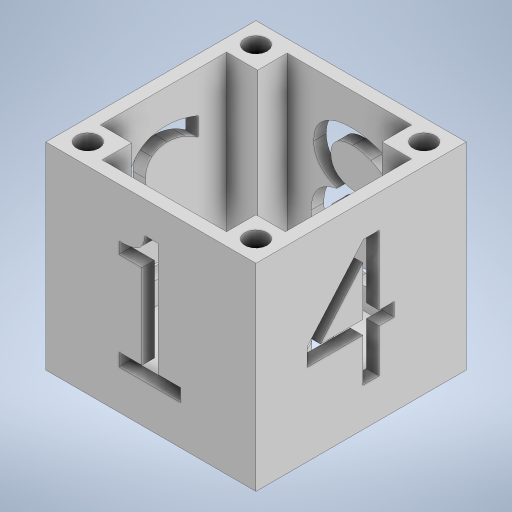
# Autodesk Inventor part: Box
Saved by Autodesk Inventor 2023 (Build 270158000, 158)
## iProperties
Created: 2023-12-17
Part Number: Box
Material: Generic
Document SubType Name: Modeling
Designer: Mustapha
Density: 1 g/cm^3
Appearance: Default
Author: Mustapha
Autodesk Inventor part; units mm, degrees
ref_plane "YZ Plane" through (0, 0, 0) normal (1, 0, 0) x (0, 1, 0)
ref_plane "XZ Plane" through (0, 0, 0) normal (0, 1, 0) x (-1, 0, 0)
ref_plane "XY Plane" through (0, 0, 0) normal (0, 0, 1) x (1, 0, 0)
sketch "Sketch1" plane through (0, 0, 0) normal (0, 1, 0) x (-1, 0, 0)
  line L0 (0, 0) -> (50, 0)
  line L1 (50, 0) -> (50, -50)
  line L2 (50, -50) -> (0, -50)
  line L3 (0, -50) -> (0, 0)
  dimension "d0" = 50
  dimension "d1" = 50
  constraints: 8 end point, 2 parallel, 1 horizontal, 1 perpendicular
  measures "d0" distance of L0.start L0.end
  measures "d1" distance of L2.end L0.start
extrude "Extrusion1" add sketch "Sketch1" along normal blind 3
sketch "Sketch2" plane through (0, 3, 0) normal (0, 1, 0) x (1, 0, 0)
  line L0 (0, 50) -> (-50, 50) projected
  line L1 (0, 50) -> (-50, 50)
  line L2 (-50, 50) -> (-50, 0)
  line L3 (-50, 0) -> (0, 0)
  line L4 (0, 0) -> (0, 50)
  line L5 (-10, 47) -> (-39.5847, 47)
  line L6 (-47, 40) -> (-47, 10)
  line L7 (-39.5847, 3) -> (-10, 3)
  line L8 (-3, 10) -> (-3, 40)
  line L9 (0, 0) -> (0, 50) projected
  line L10 (0, 50) -> (-10, 50)
  line L11 (-10, 50) -> (-10, 40)
  line L12 (-10, 40) -> (0, 40)
  line L13 (0, 40) -> (0, 50)
  line L14 (0, 25) -> (-50, 25)
  line L15 (-50, 50) -> (-50, 0) projected
  line L16 (-24.7923, 0) -> (-24.7923, 50.7224)
  line L17 (0, 0) -> (-10, 0)
  line L18 (-10, 0) -> (-10, 10)
  line L19 (-10, 10) -> (0, 10)
  line L20 (0.4153, 0) -> (-49.5847, 0)
  line L21 (-49.5847, 50) -> (-39.5847, 50)
  line L22 (-39.5847, 50) -> (-39.5847, 40)
  line L23 (-39.5847, 40) -> (-49.5847, 40)
  line L24 (-39.5847, 10) -> (-49.5847, 10)
  line L25 (-39.5847, 0) -> (-39.5847, 10)
  point P0 (-24.7923, 3)
  dimension "d10" = 3
  dimension "d11" = 3
  dimension "d12" = 3
  dimension "d13" = 3
  dimension "d14" = 10
  dimension "d15" = 10
  constraints: 46 end point, 12 symmetric about line, 8 point on line, 6 parallel, 4 perpendicular, 3 horizontal, 2 midpoint
  measures "d10" distance between parallel lines of L3 L7
  measures "d11" distance between parallel lines of L0 L5
  measures "d12" distance between parallel lines of L4 L8
  measures "d13" distance between parallel lines of L6 L2
  measures "d14" distance between parallel lines of L11 L13
  measures "d15" distance of L10.end L11.end
extrude "Extrusion2" add sketch "Sketch2" along normal blind 44 contours L4 L12 L11 L0 | L11 L5 L16 L0 | L4 L14 L8 L12 | L16 L5 L22 L0 | L4 L19 L8 L14 | L22 L23 L6 L14 L2 L0 | L4 L3 L18 L19 | L6 L24 L25 L3 L2 L14 | L16 L3 L25 L7 | L7 L18 L3 L16
sketch "Sketch3" plane through (-50, 0, 0) normal (0, 0, 1) x (1, 0, 0)
  line L0 (12.8681, 39.4555) -> (44.0571, 39.4555) construction
  line L1 (44.0571, 39.4555) -> (44.0571, 9.9644) construction
  line L2 (44.0571, 9.9644) -> (12.8681, 9.9644) construction
  line L3 (12.8681, 9.9644) -> (12.8681, 39.4555) construction
  line L4 (32.0496, 9.3582) -> (17.4143, 9.3582)
  line L5 (17.4143, 9.3582) -> (17.4143, 12.4214)
  line L6 (17.4143, 12.4214) -> (22.86, 12.4214)
  line L7 (22.86, 12.4214) -> (22.86, 32.5268)
  line L8 (22.86, 32.5268) -> (17.4143, 32.5268)
  line L9 (17.4143, 32.5268) -> (17.4143, 35.274)
  spline S0 degree 2 poles (17.4143, 35.274) (20.5018, 35.274) (23.4191, 37.0244) (23.6136, 39.4555) knots 0 0 0 1 2 2 2
  line L10 (23.6136, 39.4555) -> (26.7254, 39.4555)
  line L11 (26.7254, 39.4555) -> (26.7254, 12.4214)
  line L12 (26.7254, 12.4214) -> (32.0496, 12.4214)
  line L13 (32.0496, 12.4214) -> (32.0496, 9.3582)
  point P0 (50, 0)
  constraints: 2 other
extrude "Extrusion3" cut sketch "Sketch3" against normal blind 44
sketch "Sketch6" plane through (0, 47, 0) normal (0, 1, 0) x (1, 0, 0)
  circle A0 centre (-5, 45) radius 2.65
  line L0 (0, 0) -> (0, 50) projected
  line L1 (0, 50) -> (-50, 50) projected
  line L2 (0, 0) -> (0, 50) projected
  line L3 (0, 25) -> (-54.5112, 25)
  line L4 (0, 50) -> (-50, 50) projected
  line L5 (-25, 50) -> (-25, 0)
  circle A1 centre (-5, 5) radius 2.65
  circle A2 centre (-45, 45) radius 2.65
  circle A3 centre (-45, 5) radius 2.65
  dimension "d18" = 5
  dimension "d19" = 5
  dimension "d20" = 5.3
  dimension "d21" = 25
  constraints: 4 centre point, 4 end point, 3 symmetric about line, 2 midpoint, 1 horizontal, 1 perpendicular, 3 other
  measures "d18" distance from line of L0 A0.centre
  measures "d19" distance from line of L1 A0.centre
  measures "d20" diameter of A0
  measures "d21" distance between parallel lines of L0 L5
extrude "Extrusion4" cut sketch "Sketch6" against normal blind 5 contours A0 | A1 | A2 | A3
sketch "Sketch7" plane through (-50, 0, -50) normal (-1, 0, 0) x (0, 0, 1)
  line L0 (13.901, 39.0556) -> (42.5878, 39.0556) construction
  line L1 (42.5878, 39.0556) -> (42.5878, 7.5091) construction
  line L2 (42.5878, 7.5091) -> (13.901, 7.5091) construction
  line L3 (13.901, 7.5091) -> (13.901, 39.0556) construction
  line L4 (34.5899, 8.4235) -> (16.0891, 8.4235)
  line L5 (16.0891, 8.4235) -> (16.0891, 12.678)
  spline S0 degree 2 poles (16.0891, 12.678) (18.0826, 14.5499) (21.632, 18.0264) (23.3338, 19.8984) knots 0 0 0 1 2 2 2
  spline S1 degree 2 poles (23.3338, 19.8984) (26.7617, 23.6666) (29.2657, 28.1885) (29.2657, 30.5953) knots 0 0 0 1 2 2 2
  spline S2 degree 2 poles (29.2657, 30.5953) (29.2657, 31.8595) (28.4878, 33.7558) (27.7827, 34.3636) knots 0 0 0 1 2 2 2
  spline S3 degree 2 poles (27.7827, 34.3636) (27.0777, 34.9713) (25.2301, 35.5791) (24.1117, 35.5791) knots 0 0 0 1 2 2 2
  spline S4 degree 2 poles (24.1117, 35.5791) (23.0421, 35.5791) (20.854, 35.0443) (19.8573, 34.631) knots 0 0 0 1 2 2 2
  spline S5 degree 2 poles (19.8573, 34.631) (19.0064, 34.2906) (17.4262, 33.3182) (16.9399, 32.9778) knots 0 0 0 1 2 2 2
  line L6 (16.9399, 32.9778) -> (16.7211, 32.9778)
  line L7 (16.7211, 32.9778) -> (16.7211, 37.2566)
  spline S6 degree 2 poles (16.7211, 37.2566) (17.961, 37.8644) (22.41, 39.0556) (24.4035, 39.0556) knots 0 0 0 1 2 2 2
  spline S7 degree 2 poles (24.4035, 39.0556) (28.6093, 39.0556) (33.35, 34.6067) (33.35, 30.8141) knots 0 0 0 1 2 2 2
  spline S8 degree 2 poles (33.35, 30.8141) (33.35, 29.0394) (32.5234, 26.0734) (31.7941, 24.8093) knots 0 0 0 1 2 2 2
  spline S9 degree 2 poles (31.7941, 24.8093) (31.0647, 23.4965) (28.9497, 20.9195) (27.7827, 19.6796) knots 0 0 0 1 2 2 2
  spline S10 degree 2 poles (27.7827, 19.6796) (25.8865, 17.6132) (21.243, 13.1885) (19.8573, 11.9) knots 0 0 0 1 2 2 2
  line L8 (19.8573, 11.9) -> (34.5899, 11.9)
  line L9 (34.5899, 11.9) -> (34.5899, 8.4235)
  point P0 (50, 0)
  constraints: 2 other
extrude "Extrusion5" cut sketch "Sketch7" against normal blind 5
sketch "Sketch8" plane through (0, 0, -50) normal (0, 0, -1) x (-1, 0, 0)
  line L0 (13.682, 39.2957) -> (44.0571, 39.2957) construction
  line L1 (44.0571, 39.2957) -> (44.0571, 5.0686) construction
  line L2 (44.0571, 5.0686) -> (13.682, 5.0686) construction
  line L3 (13.682, 5.0686) -> (13.682, 39.2957) construction
  spline S0 degree 2 poles (23.9656, 35.8192) (22.8716, 35.8192) (20.7079, 35.2843) (19.6625, 34.871) knots 0 0 0 1 2 2 2
  spline S1 degree 2 poles (19.6625, 34.871) (18.6901, 34.4577) (17.2557, 33.5825) (16.6966, 33.1935) knots 0 0 0 1 2 2 2
  line L4 (16.6966, 33.1935) -> (16.4535, 33.1935)
  line L5 (16.4535, 33.1935) -> (16.4535, 37.448)
  spline S2 degree 2 poles (16.4535, 37.448) (17.7663, 38.153) (22.2638, 39.2957) (24.2817, 39.2957) knots 0 0 0 1 2 2 2
  spline S3 degree 2 poles (24.2817, 39.2957) (26.3238, 39.2957) (29.3627, 38.4691) (30.6026, 37.5939) knots 0 0 0 1 2 2 2
  spline S4 degree 2 poles (30.6026, 37.5939) (31.9154, 36.6457) (33.2768, 33.8986) (33.2768, 32.0509) knots 0 0 0 1 2 2 2
  spline S5 degree 2 poles (33.2768, 32.0509) (33.2768, 29.5712) (30.0191, 25.8273) (27.7338, 25.341) knots 0 0 0 1 2 2 2
  line L6 (27.7338, 25.341) -> (27.7338, 25.0493)
  spline S6 degree 2 poles (27.7338, 25.0493) (28.682, 24.8548) (30.8457, 23.9796) (31.7695, 23.1044) knots 0 0 0 1 2 2 2
  spline S7 degree 2 poles (31.7695, 23.1044) (32.6933, 22.2535) (33.8603, 19.5307) (33.8603, 17.5615) knots 0 0 0 1 2 2 2
  spline S8 degree 2 poles (33.8603, 17.5615) (33.8603, 15.5436) (32.4745, 12.1157) (31.2103, 10.8029) knots 0 0 0 1 2 2 2
  spline S9 degree 2 poles (31.2103, 10.8029) (29.8975, 9.4415) (26.1779, 8.0315) (23.8197, 8.0315) knots 0 0 0 1 2 2 2
  spline S10 degree 2 poles (23.8197, 8.0315) (21.5588, 8.0315) (17.1342, 9.1255) (15.6269, 9.8791) knots 0 0 0 1 2 2 2
  line L7 (15.6269, 9.8791) -> (15.6269, 14.1336)
  line L8 (15.6269, 14.1336) -> (15.9186, 14.1336)
  spline S11 degree 2 poles (15.9186, 14.1336) (17.1828, 13.2098) (21.4616, 11.508) (23.5766, 11.508) knots 0 0 0 1 2 2 2
  spline S12 degree 2 poles (23.5766, 11.508) (24.8165, 11.508) (27.2962, 12.2859) (28.1228, 13.1854) knots 0 0 0 1 2 2 2
  spline S13 degree 2 poles (28.1228, 13.1854) (28.9251, 14.085) (29.776, 16.2243) (29.776, 17.8532) knots 0 0 0 1 2 2 2
  spline S14 degree 2 poles (29.776, 17.8532) (29.776, 19.482) (28.8278, 21.5971) (27.977, 22.2049) knots 0 0 0 1 2 2 2
  spline S15 degree 2 poles (27.977, 22.2049) (27.1261, 22.8127) (24.8165, 23.2746) (23.4551, 23.2746) knots 0 0 0 1 2 2 2
  line L9 (23.4551, 23.2746) -> (21.7533, 23.2746)
  line L10 (21.7533, 23.2746) -> (21.7533, 26.6052)
  line L11 (21.7533, 26.6052) -> (23.0904, 26.6052)
  spline S16 degree 2 poles (23.0904, 26.6052) (25.7889, 26.6052) (29.1925, 29.1822) (29.1925, 31.6376) knots 0 0 0 1 2 2 2
  spline S17 degree 2 poles (29.1925, 31.6376) (29.1925, 32.7803) (28.3173, 34.4091) (27.6123, 34.8953) knots 0 0 0 1 2 2 2
  spline S18 degree 2 poles (27.6123, 34.8953) (26.8586, 35.4059) (25.011, 35.8192) (23.9656, 35.8192) knots 0 0 0 1 2 2 2
  point P0 (0, 0)
  constraints: 2 other
extrude "Extrusion6" cut sketch "Sketch8" against normal blind 5
sketch "Sketch9" plane through (0, 0, 0) normal (1, 0, 0) x (0, 0, -1)
  line L0 (11.3547, 39.1637) -> (45.4717, 39.1637) construction
  line L1 (45.4717, 39.1637) -> (45.4717, 2.8456) construction
  line L2 (45.4717, 2.8456) -> (11.3547, 2.8456) construction
  line L3 (11.3547, 2.8456) -> (11.3547, 39.1637) construction
  line L4 (32.8458, 19.4717) -> (29.272, 19.4717)
  line L5 (29.272, 19.4717) -> (29.272, 9.1637)
  line L6 (29.272, 9.1637) -> (25.4066, 9.1637)
  line L7 (25.4066, 9.1637) -> (25.4066, 19.4717)
  line L8 (25.4066, 19.4717) -> (12.157, 19.4717)
  line L9 (12.157, 19.4717) -> (12.157, 23.7018)
  line L10 (12.157, 23.7018) -> (25.5767, 39.1637)
  line L11 (25.5767, 39.1637) -> (29.272, 39.1637)
  line L12 (29.272, 39.1637) -> (29.272, 22.705)
  line L13 (29.272, 22.705) -> (32.8458, 22.705)
  line L14 (32.8458, 22.705) -> (32.8458, 19.4717)
  line L15 (25.4066, 22.705) -> (25.4066, 34.423)
  line L16 (25.4066, 34.423) -> (15.3174, 22.705)
  line L17 (15.3174, 22.705) -> (25.4066, 22.705)
  point P0 (0, 0)
  constraints: 2 other
extrude "Extrusion7" cut sketch "Sketch9" against normal blind 5
sketch "Sketch10" plane through (0, 0, 0) normal (0, -1, 0) x (1, 0, 0)
  line L0 (-36.2764, -9.4843) -> (-5.351, -9.4843) construction
  line L1 (-5.351, -9.4843) -> (-5.351, -42.6108) construction
  line L2 (-5.351, -42.6108) -> (-36.2764, -42.6108) construction
  line L3 (-36.2764, -42.6108) -> (-36.2764, -9.4843) construction
  spline S0 degree 2 poles (-15.9037, -29.9543) (-15.9037, -32.118) (-17.2894, -35.8133) (-18.5536, -37.1747) knots 0 0 0 1 2 2 2
  spline S1 degree 2 poles (-18.5536, -37.1747) (-19.8178, -38.5361) (-23.586, -40.1164) (-25.9199, -40.1164) knots 0 0 0 1 2 2 2
  spline S2 degree 2 poles (-25.9199, -40.1164) (-28.0592, -40.1164) (-32.2408, -39.1682) (-33.7724, -38.4146) knots 0 0 0 1 2 2 2
  line L4 (-33.7724, -38.4146) -> (-33.7724, -34.1601)
  line L5 (-33.7724, -34.1601) -> (-33.4806, -34.1601)
  spline S3 degree 2 poles (-33.4806, -34.1601) (-33.0187, -34.5005) (-31.2926, -35.3757) (-30.2473, -35.7647) knots 0 0 0 1 2 2 2
  spline S4 degree 2 poles (-30.2473, -35.7647) (-29.056, -36.178) (-27.0868, -36.6399) (-25.8469, -36.6399) knots 0 0 0 1 2 2 2
  spline S5 degree 2 poles (-25.8469, -36.6399) (-24.6314, -36.6399) (-22.3461, -35.7647) (-21.5195, -34.8165) knots 0 0 0 1 2 2 2
  spline S6 degree 2 poles (-21.5195, -34.8165) (-20.7659, -33.917) (-19.9879, -31.5345) (-19.9879, -29.93) knots 0 0 0 1 2 2 2
  spline S7 degree 2 poles (-19.9879, -29.93) (-19.9879, -28.3254) (-20.8631, -26.2833) (-21.6897, -25.6026) knots 0 0 0 1 2 2 2
  spline S8 degree 2 poles (-21.6897, -25.6026) (-22.5406, -24.8489) (-25.069, -24.2169) (-26.6006, -24.2169) knots 0 0 0 1 2 2 2
  spline S9 degree 2 poles (-26.6006, -24.2169) (-28.2537, -24.2169) (-31.5357, -24.7274) (-32.5325, -24.9462) knots 0 0 0 1 2 2 2
  line L6 (-32.5325, -24.9462) -> (-32.5325, -9.4843)
  line L7 (-32.5325, -9.4843) -> (-16.0738, -9.4843)
  line L8 (-16.0738, -9.4843) -> (-16.0738, -13.0094)
  line L9 (-16.0738, -13.0094) -> (-28.667, -13.0094)
  line L10 (-28.667, -13.0094) -> (-28.667, -21.0078)
  spline S10 degree 2 poles (-28.667, -21.0078) (-27.9377, -20.9105) (-26.5276, -20.8376) (-25.9442, -20.8376) knots 0 0 0 1 2 2 2
  spline S11 degree 2 poles (-25.9442, -20.8376) (-23.6346, -20.8376) (-20.4498, -21.5912) (-18.9912, -22.7096) knots 0 0 0 1 2 2 2
  spline S12 degree 2 poles (-18.9912, -22.7096) (-17.5082, -23.8279) (-15.9037, -27.2314) (-15.9037, -29.9543) knots 0 0 0 1 2 2 2
  point P0 (0, 0)
  constraints: 2 other
extrude "Extrusion8" cut sketch "Sketch10" against normal blind 5
equation "\"d11\" = d10"
equation "\"d12\" = d10"
equation "\"d13\" = d10"
body "Solid1"
